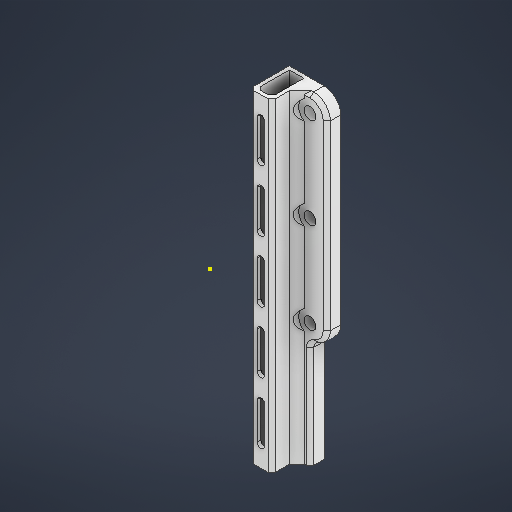
# Autodesk Inventor part: CNC-028-WireTrack1
Saved by Autodesk Inventor 2026.2 (Build 302298000, 298)
## iProperties
Created: 2026-06-26
Part Number: CNC-028-WireTrack1
Material: ABS Plastic
Document SubType Name: Modeling
Designer: Kenji
Density: 1.06 g/cm^3
Appearance: Smooth - White
Author: Kenji
Autodesk Inventor part; units mm, degrees
ref_plane "YZ Plane" through (0, 0, 0) normal (1, 0, 0) x (0, 1, 0)
ref_plane "XZ Plane" through (0, 0, 0) normal (0, 1, 0) x (-1, 0, 0)
ref_plane "XY Plane" through (0, 0, 0) normal (0, 0, 1) x (1, 0, 0)
ref_plane "Work Plane1" through (0, 0, 0) normal (0, 0, 1) x (1, 0, 0)
sketch "Sketch1" plane through (0, 0, 0) normal (0, 0, 1) x (1, 0, 0)
  circle A0 centre (50, -17.5) radius 2.6 projected
  circle A1 centre (50, 22.5) radius 2.6 projected
  circle A2 centre (50, 62.5) radius 2.6 projected
  circle A3 centre (50, -17.5) radius 7.3625 construction
  circle A4 centre (50, 22.5) radius 7.3625 construction
  circle A5 centre (50, 62.5) radius 7.3625 construction
  line L0 (50, -24.8625) -> (42.6375, -24.8625)
  line L1 (42.6375, -24.8625) -> (42.6375, 69.8625)
  line L2 (42.6375, 69.8625) -> (50, 69.8625)
  line L3 (57.3625, -17.5) -> (57.3625, 62.5)
  arc A6 (50, -24.8625) -> (57.3625, -17.5) centre (50, -17.5) ccw
  arc A7 (57.3625, 62.5) -> (50, 69.8625) centre (50, 62.5) ccw
  circle A8 centre (50, -17.5) radius 5 construction
  point P0 (0, 0)
  dimension "d0" = 4.7625
  dimension "d1" = 10
  constraints: 8 end point, 8 point on circle, 6 centre point, 4 equal radius, 4 tangent, 3 coincident, 2 perpendicular, 1 horizontal, 1 vertical
  measures "d0" radial gap between concentric circles of A3 A0
  measures "d1" diameter of A8
extrude "Extrusion1" add sketch "Sketch1" along normal blind 6.175
sketch "Sketch2" plane through (0, 0, 6.175) normal (0, 0, 1) x (1, 0, 0)
  line L0 (42.6375, 69.8625) -> (42.6375, -24.8625) projected
  circle A0 centre (50, -17.5) radius 2.6 projected
  circle A1 centre (50, -17.5) radius 5 construction
  line L1 (42.6375, -24.8625) -> (50, -24.8625) construction
  line L2 (44.225, -24.8625) -> (44.225, 69.8625)
  line L3 (42.6375, 69.8625) -> (44.225, 69.8625)
  line L4 (42.6375, -24.8625) -> (44.225, -24.8625)
  point P0 (0, 0)
  dimension "d4" = 10
  dimension "d34" = 1.5875
  constraints: 6 end point, 1 centre point, 1 coincident, 1 collinear, 1 horizontal, 1 point on line, 1 vertical
  measures "d4" diameter of A1
  measures "d34" distance between parallel lines of L2 L0
ref_plane "Work Plane2" through (40.2375, 90.7678, 31.75) normal (0, 0, 1) x (1, 0, 0)
extrude "Extrusion2" add sketch "Sketch2" along normal blind 9.525 contours L3 L2 L4 L0
chamfer "Chamfer1" distance 3.175 angle 45 1 edges at (44.225, 22.5, 6.175)
sketch "Sketch3" plane through (0, 0, 6.175) normal (0, 0, 1) x (1, 0, 0)
  circle A0 centre (50, -17.5) radius 2.6 projected
  circle A1 centre (50, -17.5) radius 5
  circle A2 centre (50, 22.5) radius 2.6 projected
  circle A3 centre (50, 62.5) radius 2.6 projected
  circle A4 centre (50, 22.5) radius 5
  circle A5 centre (50, 62.5) radius 5
  point P0 (0, 0)
  point P1 (48.175, -15.6481)
  point P2 (48.175, -19.3519)
  point P3 (48.175, 24.3519)
  point P4 (48.175, 20.6481)
  point P5 (48.175, 64.3519)
  point P6 (48.175, 60.6481)
  dimension "d10" = 10
  constraints: 3 centre point, 3 coincident, 2 equal radius
  measures "d10" diameter of A1
extrude "Extrusion3" cut sketch "Sketch3" along normal blind 25.4 contours A0 | A1 | A2 | A3 | A4 | A5
sketch "Sketch4" plane through (0, 0, 15.7) normal (0, 0, 1) x (1, 0, 0)
  line L0 (42.6375, -24.8625) -> (44.225, -24.8625) projected
  line L1 (44.225, -24.8625) -> (34.7, -24.8625)
  line L2 (34.7, -24.8625) -> (34.7, 69.8625)
  line L3 (34.7, 69.8625) -> (44.225, 69.8625)
  line L4 (44.225, 69.8625) -> (44.225, -24.8625)
  line L5 (44.225, 69.8625) -> (42.6375, 69.8625) projected
  line L6 (34.7, -24.8625) -> (36.2875, -24.8625)
  line L7 (36.2875, -24.8625) -> (36.2875, 69.8625)
  line L8 (36.2875, 69.8625) -> (34.7, 69.8625)
  line L9 (34.7, 69.8625) -> (34.7, -24.8625)
  line L10 (42.6375, 69.8625) -> (42.6375, -24.8625) projected
  point P0 (0, 0)
  dimension "d13" = 9.525
  dimension "d15" = 1.5875
  dimension "d16" = 1.5875
  constraints: 16 end point, 4 parallel, 2 collinear, 2 horizontal, 2 perpendicular
  measures "d13" distance between parallel lines of L4 L2
  measures "d15" distance between parallel lines of L7 L2
  measures "d16" distance between parallel lines of L4 L10
ref_plane "Work Plane3" through (-55.775, -68.275, 0) normal (0, 0, 1) x (1, 0, 0)
extrude "Extrusion4" add sketch "Sketch4" against normal up to surface (15.7 mm away) contours L1 L2 L3 L7
sketch "Sketch5" plane through (0, 0, 15.7) normal (0, 0, 1) x (1, 0, 0)
  line L0 (34.7, -24.8625) -> (34.7, 69.8625) projected
  line L1 (50, 69.8625) -> (42.6375, 69.8625) projected
  line L2 (34.7, -24.8625) -> (44.225, -24.8625)
  line L3 (44.225, -24.8625) -> (44.225, 69.8625)
  line L4 (44.225, 69.8625) -> (34.7, 69.8625)
  line L5 (34.7, 69.8625) -> (34.7, -24.8625)
  line L6 (44.225, -24.8625) -> (44.225, 69.8625) projected
  point P0 (0, 0)
  constraints: 8 end point, 2 parallel, 1 collinear, 1 horizontal, 1 perpendicular, 1 point on line
extrude "Extrusion5" add sketch "Sketch5" along normal blind 1.5875
chamfer "Chamfer2" distance 1.5875 angle 45 4 edges at (44.225, 22.5, 17.2875) (34.7, 22.5, 17.2875) (36.2875, 22.5, 15.7) (42.6375, 22.5, 15.7)
sketch "Sketch7" plane through (42.6375, -24.8625, 0) normal (0, -1, 0) x (1, 0, 0)
  point P0 (-42.6375, 0)
sketch "Sketch8" plane through (42.6375, -24.8625, 0) normal (0, -1, 0) x (1, 0, 0)
  line L0 (-7.9375, 15.7) -> (-6.35, 17.2875) projected
  line L1 (-7.9375, 0) -> (-7.9375, 15.7) projected
  line L2 (-6.35, 0) -> (-7.9375, 0) projected
  line L3 (-6.35, 14.1125) -> (-6.35, 0) projected
  line L4 (-4.7625, 15.7) -> (-6.35, 14.1125) projected
  line L5 (-4.7625, 15.7) -> (-1.5875, 15.7) projected
  line L6 (0, 14.1125) -> (-1.5875, 15.7) projected
  line L7 (0, 0) -> (0, 14.1125) projected
  line L8 (0, 0) -> (7.3625, 0) projected
  line L9 (7.3625, 0) -> (7.3625, 6.175) projected
  line L10 (4.7625, 6.175) -> (7.3625, 6.175) projected
  line L11 (1.5875, 9.35) -> (4.7625, 6.175) projected
  line L12 (1.5875, 9.35) -> (1.5875, 15.7) projected
  line L13 (0, 17.2875) -> (1.5875, 15.7) projected
  line L14 (-6.35, 17.2875) -> (0, 17.2875) projected
  point P0 (-42.6375, 0)
ref_plane "Work Plane4" through (-290, -72.5, -10.037) normal (0, -1, 0) x (1, 0, 0)
extrude "Extrusion7" add sketch "Sketch8" along normal up to surface (47.6375 mm away)
fillet "Fillet1" radius 3.175 1 edges at (50, -24.8625, 3.0875)
sketch "Sketch9" plane through (0, 0, 17.2875) normal (0, 0, 1) x (1, 0, 0)
  line L0 (36.2875, 69.8625) -> (36.2875, -72.5) projected
  line L1 (42.6375, 69.8625) -> (42.6375, -72.5) projected
  line L2 (39.4625, -63.3595) -> (39.4625, -47.1256) construction
  line L3 (41.05, -63.3595) -> (41.05, -47.1256)
  line L4 (37.875, -47.1256) -> (37.875, -63.3595)
  arc A0 (37.875, -63.3595) -> (41.05, -63.3595) centre (39.4625, -63.3595) ccw
  arc A1 (41.05, -47.1256) -> (37.875, -47.1256) centre (39.4625, -47.1256) ccw
  line L5 (36.2875, -72.5) -> (42.6375, -72.5) projected
  line L6 (39.4625, -36.3976) -> (39.4625, -20.1637) construction
  line L7 (41.05, -36.3976) -> (41.05, -20.1637)
  line L8 (37.875, -20.1637) -> (37.875, -36.3976)
  arc A2 (37.875, -36.3976) -> (41.05, -36.3976) centre (39.4625, -36.3976) ccw
  arc A3 (41.05, -20.1637) -> (37.875, -20.1637) centre (39.4625, -20.1637) ccw
  line L9 (39.4625, -9.4357) -> (39.4625, 6.7982) construction
  line L10 (41.05, -9.4357) -> (41.05, 6.7982)
  line L11 (37.875, 6.7982) -> (37.875, -9.4357)
  arc A4 (37.875, -9.4357) -> (41.05, -9.4357) centre (39.4625, -9.4357) ccw
  arc A5 (41.05, 6.7982) -> (37.875, 6.7982) centre (39.4625, 6.7982) ccw
  line L12 (39.4625, 17.5262) -> (39.4625, 33.7601) construction
  line L13 (41.05, 17.5262) -> (41.05, 33.7601)
  line L14 (37.875, 33.7601) -> (37.875, 17.5262)
  arc A6 (37.875, 17.5262) -> (41.05, 17.5262) centre (39.4625, 17.5262) ccw
  arc A7 (41.05, 33.7601) -> (37.875, 33.7601) centre (39.4625, 33.7601) ccw
  line L15 (39.4625, 44.4881) -> (39.4625, 60.722) construction
  line L16 (41.05, 44.4881) -> (41.05, 60.722)
  line L17 (37.875, 60.722) -> (37.875, 44.4881)
  arc A8 (37.875, 44.4881) -> (41.05, 44.4881) centre (39.4625, 44.4881) ccw
  arc A9 (41.05, 60.722) -> (37.875, 60.722) centre (39.4625, 60.722) ccw
  line L18 (42.6375, 69.8625) -> (36.2875, 69.8625) projected
  point P0 (0, 0)
  point P1 (39.4625, -55.2425)
  point P2 (39.4625, -72.5)
  point P3 (39.4625, -64.947)
  point P4 (39.4625, -72.5)
  point P5 (39.4625, -28.2806)
  point P6 (39.4625, -1.3187)
  point P7 (39.4625, 25.6431)
  point P8 (39.4625, 52.605)
  point P9 (39.4625, 69.8625)
  point P10 (39.4625, 62.3095)
  point P11 (39.4625, -37.9851)
  point P12 (39.4625, -45.5381)
  point P13 (39.4625, -11.0232)
  point P14 (39.4625, -18.5762)
  point P15 (39.4625, 15.9387)
  point P16 (39.4625, 8.3857)
  point P17 (39.4625, 42.9006)
  point P18 (39.4625, 35.3476)
  dimension "d38" = 1.5875
  dimension "d39" = 7.553
  dimension "d40" = 16.2339
  dimension "d41" = 7.553
  dimension "d46" = 7.553
  dimension "d47" = 7.553
  dimension "d48" = 7.553
  dimension "d49" = 7.553
  constraints: 40 end point, 30 point on circle, 20 tangent, 10 centre point, 8 midpoint, 7 point on line, 5 collinear, 5 parallel, 4 equal radius, 2 vertical
  measures "d38" distance between parallel lines of L0 L4
  measures "d39" distance of point (39.462, -64.947) point (39.462, -72.5)
  measures "d40" distance of L2.end L2.start
  measures "d41" distance of point (39.462, 69.862) point (39.462, 62.309)
  measures "d46" distance of point (39.462, -37.985) point (39.462, -45.538)
  measures "d47" distance of point (39.462, -11.023) point (39.462, -18.576)
  measures "d48" distance of point (39.462, 15.939) point (39.462, 8.386)
  measures "d49" distance of point (39.462, 42.901) point (39.462, 35.348)
extrude "Extrusion8" cut sketch "Sketch9" against normal through all contours A0 L4 A1 L3 | A2 L8 A3 L7 | A4 L11 A5 L10 | A6 L14 A7 L13 | A8 L17 A9 L16
sketch "Sketch10" plane through (42.6375, 69.8625, 0) normal (0, 1, 0) x (1, 0, 0)
  line L0 (-6.35, -1.5875) -> (0, -1.5875)
  line L1 (-6.35, -14.1125) -> (-6.35, 0) projected
  line L2 (0, 0) -> (0, -14.1125) projected
  line L3 (26.1975, 0) -> (-54.11, 0) projected
  point P0 (-42.6375, 0)
  dimension "d53" = 1.5875
  constraints: 2 end point, 2 point on line
  measures "d53" distance between parallel lines of L0 L3
extrude "Extrusion9" add sketch "Sketch10" against normal up to surface (142.3625 mm away)
chamfer "Chamfer3" distance 1.5875 angle 45 6 edges at (50, -50.0239, 6.175) (50.6139, -25.6712, 6.175) (55.9388, -21.8517, 6.175) (57.3625, 22.5, 6.175) (55.2061, 67.7061, 6.175) (48.6999, 69.8625, 6.175)
sketch "Sketch11" plane through (36.2875, -72.5, 1.5875) normal (0, 0, 1) x (1, 0, 0)
  line L0 (1.5875, 63.0643) -> (1.5875, 79.2982) projected
  arc A0 (4.7625, 79.2982) -> (1.5875, 79.2982) centre (3.175, 79.2982) ccw projected
  line L1 (4.7625, 79.2982) -> (4.7625, 63.0643) projected
  arc A1 (1.5875, 63.0643) -> (4.7625, 63.0643) centre (3.175, 63.0643) ccw projected
  line L2 (1.5875, 90.0262) -> (1.5875, 106.2601) projected
  arc A2 (4.7625, 106.2601) -> (1.5875, 106.2601) centre (3.175, 106.2601) ccw projected
  line L3 (4.7625, 106.2601) -> (4.7625, 90.0262) projected
  arc A3 (1.5875, 90.0262) -> (4.7625, 90.0262) centre (3.175, 90.0262) ccw projected
  line L4 (1.5875, 36.1024) -> (1.5875, 52.3363) projected
  arc A4 (4.7625, 52.3363) -> (1.5875, 52.3363) centre (3.175, 52.3363) ccw projected
  line L5 (4.7625, 52.3363) -> (4.7625, 36.1024) projected
  arc A5 (1.5875, 36.1024) -> (4.7625, 36.1024) centre (3.175, 36.1024) ccw projected
  line L6 (1.5875, 116.9881) -> (1.5875, 133.222) projected
  arc A6 (4.7625, 133.222) -> (1.5875, 133.222) centre (3.175, 133.222) ccw projected
  line L7 (4.7625, 133.222) -> (4.7625, 116.9881) projected
  arc A7 (1.5875, 116.9881) -> (4.7625, 116.9881) centre (3.175, 116.9881) ccw projected
  line L8 (1.5875, 9.1405) -> (1.5875, 25.3744) projected
  arc A8 (4.7625, 25.3744) -> (1.5875, 25.3744) centre (3.175, 25.3744) ccw projected
  line L9 (4.7625, 25.3744) -> (4.7625, 9.1405) projected
  arc A9 (1.5875, 9.1405) -> (4.7625, 9.1405) centre (3.175, 9.1405) ccw projected
  line L10 (0, 142.3625) -> (0, 0) projected
  line L11 (0, 0) -> (6.35, 0) projected
  line L12 (6.35, 142.3625) -> (6.35, 0) projected
  line L13 (6.35, 142.3625) -> (0, 142.3625) projected
  point P0 (-36.2875, 72.5)
extrude "Extrusion10" cut sketch "Sketch11" against normal blind 25.4 contours L0 A0 L1 A1 | L2 A2 L3 A3 | L4 A4 L5 A5 | L6 A6 L7 A7 | L8 A8 L9 A9
equation "\"d15\" = d16"
equation "\"d41\" = d39"
equation "\"d46\" = d39"
equation "\"d47\" = d46"
equation "\"d48\" = d47"
equation "\"d49\" = d48"
body "Solid1"
